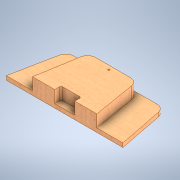
# Autodesk Inventor part: Pont arriere
Saved by Autodesk Inventor 2021 (Build 250183000, 183)
## iProperties
Created: 2021-01-15
Part Number: Pont arriere
Material: Bois (Cerisier)
Document SubType Name: Modeling
Designer: dimercur
Density: 0.63 g/cm^3
Appearance: Cerisier - Faible lustre naturel
Author: dimercur
Autodesk Inventor part; units mm, degrees
ref_plane "YZ Plane" through (0, 0, 0) normal (1, 0, 0) x (0, 1, 0)
ref_plane "XZ Plane" through (0, 0, 0) normal (0, 1, 0) x (-1, 0, 0)
ref_plane "XY Plane" through (0, 0, 0) normal (0, 0, 1) x (1, 0, 0)
sketch "Esquisse1" plane through (0, 0, 0) normal (0, 1, 0) x (-1, 0, 0)
  line L0 (-70.5281, 61.3918) -> (-58.0281, -1.6082)
  line L1 (-58.0281, -1.6082) -> (61.9719, -1.6082)
  line L2 (61.9719, -1.6082) -> (74.4719, 61.3918)
  line L3 (74.4719, 61.3918) -> (-70.5281, 61.3918)
  dimension "d2" = 145
  dimension "d3" = 120
  dimension "d4" = 63
  dimension "d5" = 12.5
  constraints: 8 end point, 1 horizontal, 1 parallel
  measures "d2" distance of L2.end L0.start
  measures "d3" distance of L0.end L1.end
  measures "d4" distance between parallel lines of L1 L3
  measures "d5" horizontal distance of L0.end L0.start
extrude "Extrusion1" add sketch "Esquisse1" along normal blind 5
sketch "Esquisse2" plane through (0, 5, 0) normal (0, 1, 0) x (1, 0, 0)
  line L0 (-74.4719, -61.3918) -> (70.5281, -61.3918) projected
  line L1 (38.0281, -61.3918) -> (28.0281, -1.3918)
  line L2 (28.0281, -1.3918) -> (-31.9719, -1.3918)
  line L3 (-31.9719, -1.3918) -> (-41.9719, -61.3918)
  line L4 (-41.9719, -61.3918) -> (-14.4719, -61.3918)
  line L5 (-14.4719, -61.3918) -> (-14.4719, -53.3918)
  line L6 (-14.4719, -53.3918) -> (10.5281, -53.3918)
  line L7 (10.5281, -53.3918) -> (10.5281, -61.3918)
  line L8 (10.5281, -61.3918) -> (38.0281, -61.3918)
  point P0 (0, 0)
  dimension "d8" = 60
  dimension "d9" = 80
  dimension "d10" = 60
  dimension "d11" = 10
  dimension "d12" = 145
  dimension "d13" = 32.5
  dimension "d14" = 25
  dimension "d15" = 27.5
  dimension "d16" = 8
  constraints: 16 end point, 4 perpendicular, 3 point on line, 1 horizontal, 1 parallel
  measures "d8" vertical distance of L1.end L1.start
  measures "d9" distance of L3.end L1.start
  measures "d10" distance of L1.end L2.end
  measures "d11" horizontal distance of L1.end L1.start
  measures "d12" distance of L0.start L0.end
  measures "d13" distance of L0.end L1.start
  measures "d14" distance of L5.end L6.end
  measures "d15" distance of L7.end L1.start
  measures "d16" distance of L4.end L5.end
extrude "Extrusion2" add sketch "Esquisse2" along normal blind 15 contours L3 L2 L1 L0 L7 L6 L5
fillet "Congé1" radius 10 4 edges at (58.0281, 2.5, -1.6082) (-61.9719, 2.5, -1.6082) (-31.9719, 12.5, 1.3918) (28.0281, 12.5, 1.3918)
fillet "Congé2" radius 2 2 edges at (10.5281, 12.5, 53.3918) (-14.4719, 12.5, 53.3918)
sketch "Esquisse3" plane through (0, 20, 0) normal (0, 1, 0) x (1, 0, 0)
  circle A0 centre (-1.9719, -6.3918) radius 1
  line L0 (-14.4719, -61.3918) -> (-14.4719, -55.3918) projected
  line L1 (10.5281, -55.3918) -> (10.5281, -61.3918) projected
  line L2 (19.5569, -1.3918) -> (-23.5006, -1.3918) projected
  point P0 (0, 0)
  dimension "d21" = 2
  dimension "d22" = 25
  dimension "d23" = 12.5
  dimension "d24" = 5
  constraints: 1 centre point
  measures "d21" diameter of A0
  measures "d22" distance between parallel lines of L0 L1
  measures "d23" distance from line of A0.centre L1
  measures "d24" distance from line of L2 A0.centre
extrude "Extrusion3" cut sketch "Esquisse3" against normal blind 10
sketch "Esquisse4" plane through (19.5569, 5, 1.3918) normal (0, 0, -1) x (-1, 0, 0)
  circle A0 centre (21.5287, 7.5) radius 4
  line L0 (-30.2605, 0) -> (73.3179, 0) projected
  line L1 (0, 15) -> (43.0575, 15) projected
  line L2 (61.5287, 0) -> (61.5287, 15) projected
  line L3 (-18.4713, 0) -> (-18.4713, 15) projected
  point P0 (19.5569, -5)
  dimension "d27" = 8
  dimension "d28" = 15
  dimension "d29" = 80
  dimension "d30" = 40
  dimension "d31" = 7.5
  constraints: 1 centre point
  measures "d27" diameter of A0
  measures "d28" distance between parallel lines of L0 L1
  measures "d29" distance between parallel lines of L2 L3
  measures "d30" distance from line of L3 A0.centre
  measures "d31" distance from line of L1 A0.centre
extrude "Extrusion4" cut sketch "Esquisse4" against normal blind 30
equation "\"d5\" = -0.5 * d3 + 0.5 * d2"
equation "\"d11\" = -0.5 * d10 + 0.5 * d9"
equation "\"d13\" = -0.5 * d9 + 0.5 * d12"
equation "\"d15\" = -0.5 * d14 + 0.5 * d9"
equation "\"d23\" = 0.5 * d22"
equation "\"d30\" = 0.5 * d29"
equation "\"d31\" = 0.5 * d28"
